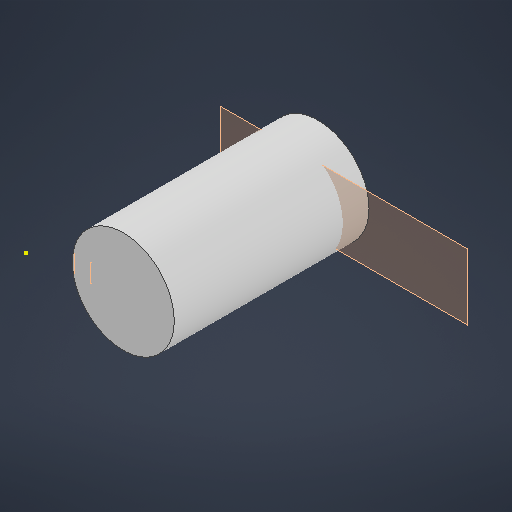
# Autodesk Inventor part: rim-v1
Saved by Autodesk Inventor 2026.2 (Build 302298010, 298A)
## iProperties
Created: 2026-05-11
Part Number: rim-v1
Material: Generic
Document SubType Name: Modeling
Designer: karol
Density: 1 g/cm^3
Appearance: Default
Author: karol
Autodesk Inventor part; units mm, degrees
ref_plane "YZ Plane" through (0, 0, 0) normal (1, 0, 0) x (0, 1, 0)
ref_plane "XZ Plane" through (0, 0, 0) normal (0, 1, 0) x (-1, 0, 0)
ref_plane "XY Plane" through (0, 0, 0) normal (0, 0, 1) x (1, 0, 0)
ref_plane "Work Plane1" through (0, 0, 0.5) normal (0, 0, 1) x (1, 0, 0)
sketch "Sketch1" plane through (0, 0, 0.5) normal (0, 0, 1) x (1, 0, 0)
  arc A0 (13, 1.882) -> (13, 4.118) centre (14, 3) ccw projected
  arc A1 (13, 1.882) -> (13, 4.118) centre (14, 3) ccw projected
  line L0 (13, 4.118) -> (13, 1.882) projected
  circle A2 centre (14, 3) radius 6
  circle A3 centre (14, 3) radius 4
  circle A4 centre (14, 3) radius 1.7
  line L1 (12.7, 1.9046) -> (12.7, 4.0954)
  point P0 (0, 0)
  dimension "d0" = 12
  dimension "d1" = 8
  dimension "d2" = 0.2
  dimension "d3" = 0.3
  constraints: 3 centre point, 3 coincident, 2 end point, 2 point on circle, 1 parallel, 1 vertical
  measures "d0" diameter of A2
  measures "d1" diameter of A3
  measures "d2" radial gap between concentric circles of A0 A4
  measures "d3" distance between parallel lines of L0 L1
extrude "Extrusion1" add sketch "Sketch1" along normal blind 21.5 contours A3 | L1 A4 picked at (12.5667, 3)
ref_plane "Work Plane2" through (14, 3, 18) normal (0, 0, 1) x (1, 0, 0)
sketch "Sketch2" plane through (14, 3, 18) normal (0, 0, 1) x (1, 0, 0)
  circle A0 centre (0, 0) radius 4 projected
  arc A1 (-1.3, -1.0954) -> (-1.3, 1.0954) centre (0, 0) ccw projected
  line L0 (-1.3, -1.0954) -> (-1.3, 1.0954) projected
  circle A2 centre (0, 0) radius 3
  point P0 (-14, -3)
  dimension "d7" = 6
  constraints: 1 centre point, 1 coincident
  measures "d7" diameter of A2
extrude "Extrusion2" cut sketch "Sketch2" against normal blind 2 contours A0
ref_plane "Work Plane3" through (9.7, 1.9046, 0.5) normal (1, 0, 0) x (0, 0, -1)
sketch "Sketch3" plane through (9.7, 1.9046, 0.5) normal (1, 0, 0) x (0, 0, -1)
  circle A0 centre (-2.5, 1) radius 1.42
  line L0 (-21.5, 0) -> (-21.5, 2.1909) projected
  point P0 (0.5, -1.9046)
  dimension "d11" = 2.84
  dimension "d12" = 1
  dimension "d15" = 19
  constraints: 1 centre point
  measures "d11" diameter of A0
  measures "d12" vertical distance of L0.start A0.centre
  measures "d15" distance from line of L0 A0.centre
extrude "Extrusion3" cut sketch "Sketch3" along normal blind 3
chamfer "Chamfer1" distance 0.25 angle 45 1 edges at (10.0014, 2.8952, 4.42)
ref_plane "Work Plane4" through (14, 3, 13) normal (0, 0, 1) x (1, 0, 0)
sketch "Sketch4" plane through (14, 3, 13) normal (0, 0, 1) x (1, 0, 0)
  circle A0 centre (0, 0) radius 4 projected
  circle A1 centre (0, 0) radius 4 projected
  circle A2 centre (0, 0) radius 3 projected
  point P0 (-14, -3)
extrude "Extrusion4" cut sketch "Sketch4" against normal blind 2
sketch "Sketch5" plane through (14, 3, 22) normal (0, 0, 1) x (1, 0, 0)
  point P0 (-14, -3)
sketch "Sketch6" plane through (14, 3, 22) normal (0, 0, 1) x (1, 0, 0)
  circle A0 centre (0, 0) radius 3 projected
  circle A1 centre (0, 0) radius 6
  circle A2 centre (0, 0) radius 6.8
  point P0 (-14, -3)
  dimension "d22" = 12
  dimension "d23" = 13.6
  constraints: 2 centre point, 2 coincident
  measures "d22" diameter of A1
  measures "d23" diameter of A2
extrude "Extrusion5" add sketch "Sketch6" against normal blind 25 contours A2
extrude "Extrusion6" add sketch "Sketch6" along normal blind 1 contours A0 | A1 | A2
ref_plane "Płaszczyzna konstrukcyjna5" through (7.5, 1.9046, 0.5) normal (1, 0, 0) x (0, 0, -1)
sketch "Szkic7" plane through (7.5, 1.9046, 0.5) normal (1, 0, 0) x (0, 0, -1)
  spline S0 degree 5 poles (-1.08, 1) (-1.08, 1.1328) (-1.0956, 1.2653) (-1.1264, 1.3939) (-1.171, 1.516) (-1.2831, 1.7427) (-1.3509, 1.8479) (-1.4285, 1.9436) (-1.5144, 2.0293) (-1.7594, 2.2271) (-1.9301, 2.3223) (-2.1149, 2.3872) (-2.3075, 2.42) (-2.7383, 2.42) (-2.9765, 2.3695) (-3.2003, 2.2706) (-3.3982, 2.1268) (-3.7238, 1.7607) (-3.8506, 1.5395) (-3.9338, 1.2774) (-3.9442, 0.9995) (-3.8575, 0.5323) (-3.7802, 0.3361) (-3.6722, 0.1617) (-3.54, 0.0138) (-3.2367, -0.2294) (-3.0658, -0.3241) (-2.8802, -0.3887) (-2.6863, -0.421) (-2.24, -0.4186) (-1.989, -0.3607) (-1.7559, -0.2492) (-1.5536, -0.0895) (-1.2778, 0.2543) (-1.1845, 0.4171) (-1.1146, 0.6037) (-1.08, 0.8006) (-1.08, 1) knots 0 0 0 0 0 0 0.068925 0.068925 0.068925 0.068925 0.13785 0.13785 0.13785 0.13785 0.250096 0.250096 0.250096 0.250096 0.389026 0.389026 0.389026 0.389026 0.527577 0.527577 0.527577 0.527577 0.639316 0.639316 0.639316 0.639316 0.751056 0.751056 0.751056 0.751056 0.896518 0.896518 0.896518 0.896518 1 1 1 1 1 1 projected
  point P0 (0.5, -1.9046)
  constraints: 1 other
extrude "Wyciągnięcie proste7" cut sketch "Szkic7" along normal mid plane 2
body "Solid1"
